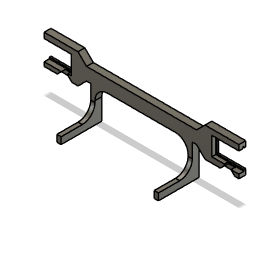
Camera Mount v7 (Autodesk Fusion 360 design; units mm, degrees)
Autodesk Fusion 360 part; units mm, degrees
sketch "Sketch1" plane through (0, 0, 0) normal (0, 0, 1) x (1, 0, 0)
  line L0 (0, 0) -> (-150, 0)
  line L1 (-150, 0) -> (-150, 15)
  line L2 (-150, 15) -> (0, 15)
  line L3 (0, 15) -> (0, 0)
  line L4 (-150, -10) -> (-158, -10)
  line L5 (-158, -10) -> (-158, 25)
  line L6 (-158, 25) -> (-150, 25)
  line L7 (-150, 25) -> (-150, -10)
  line L8 (-158, -5) -> (-188, -5)
  line L9 (-188, -5) -> (-188, 20)
  line L10 (-188, 20) -> (-158, 20)
  line L11 (-158, 20) -> (-158, -5)
  line L12 (-158, -10) -> (-190, -10)
  line L13 (-190, -10) -> (-190, -3.5)
  line L14 (-190, -3.5) -> (-158, -3.5)
  line L15 (-158, -3.5) -> (-158, -10)
  line L16 (-158, 25) -> (-190, 25)
  line L17 (-190, 25) -> (-190, 18.5)
  line L18 (-190, 18.5) -> (-158, 18.5)
  line L19 (-158, 18.5) -> (-158, 25)
  line L20 (0, 25) -> (8, 25)
  line L21 (8, 25) -> (8, -10)
  line L22 (8, -10) -> (0, -10)
  line L23 (0, -10) -> (0, 25)
  line L24 (8, 25) -> (40, 25)
  line L25 (40, 25) -> (40, 18.5)
  line L26 (40, 18.5) -> (8, 18.5)
  line L27 (8, 18.5) -> (8, 25)
  line L28 (8, -10) -> (40, -10)
  line L29 (40, -10) -> (40, -3.5)
  line L30 (40, -3.5) -> (8, -3.5)
  line L31 (8, -3.5) -> (8, -10)
  dimension "d1" = 150
  dimension "d2" = 15
  dimension "d3" = 8
  dimension "d4" = 35
  dimension "d5" = 10
  dimension "d6" = 30
  dimension "d7" = 25
  dimension "d8" = 5
  dimension "d9" = 6.5
  dimension "d10" = 32
  dimension "d11" = 32
  dimension "d12" = 6.5
  dimension "d13" = 8
  dimension "d14" = 35
  dimension "d15" = 10
  dimension "d16" = 32
  dimension "d17" = 6.5
  dimension "d18" = 32
  dimension "d19" = 6.5
  constraint horizontal L0
  constraint vertical L1
  constraint horizontal L2
  constraint vertical L3
  constraint coincident L0.start L3.end
  constraint horizontal L4
  constraint vertical L5
  constraint horizontal L6
  constraint vertical L7
  constraint horizontal L8
  constraint vertical L9
  constraint horizontal L10
  constraint vertical L11
  constraint coincident L5 L8.start
  constraint horizontal L12
  constraint vertical L13
  constraint horizontal L14
  constraint vertical L15
  constraint horizontal L16
  constraint vertical L17
  constraint horizontal L18
  constraint vertical L19
  constraint horizontal L20
  constraint vertical L21
  constraint horizontal L22
  constraint vertical L23
  constraint horizontal L24
  constraint vertical L25
  constraint horizontal L26
  constraint vertical L27
  constraint horizontal L28
  constraint vertical L29
  constraint horizontal L30
  constraint vertical L31
  measures "d1" distance of L0.start L0.end
  measures "d2" distance of L0.end L1.end
  measures "d3" distance of L4.start L4.end
  measures "d4" distance of L4.start L6.end
  measures "d5" distance of L2 L6
  measures "d6" distance of L8.start L8.end
  measures "d7" distance of L8.start L10.end
  measures "d8" distance of L2 L10
  measures "d9" distance of L4.end L14.end
  measures "d10" distance of L4.end L12.end
  measures "d11" distance of L5.end L16.end
  measures "d12" distance of L5.end L18.end
  measures "d13" distance of L20.start L20.end
  measures "d14" distance of L20.start L22.end
  measures "d15" distance of L2 L20
  measures "d16" distance of L20.end L24.end
  measures "d17" distance of L20.end L26.end
  measures "d18" distance of L21.end L28.end
  measures "d19" distance of L21.end L30.end
extrude "Extrude1" add sketch "Sketch1" along normal blind 8 contours L0 L1 L2 L3 L7 L23 | L3 L20 L21 L22 L23 L27 L31 | L1 L4 L5 L6 L7 L11 L15 L19 | L21 L28 L29 L30 L31 | L5 L8 L9 L12 L13 L14 L15 | L21 L24 L25 L26 L27 | L5 L9 L10 L16 L17 L18 L19 | L5 L8 L9 L11 L14 L15 | L5 L9 L10 L11 L18 L19
sketch "Sketch2" plane through (-190, 0, 0) normal (-1, 0, 0) x (0, 0, 1)
  line L0 (0, -3.5) -> (0, -10)
  line L1 (0, -10) -> (8, -10)
  line L2 (8, -10) -> (8, -3.5)
  line L3 (8, -3.5) -> (0, -3.5)
  line L4 (2, -3.5) -> (3.25, -3.5)
  line L5 (3.25, -3.5) -> (3.25, -5.25)
  line L6 (3.25, -5.25) -> (2, -5.25)
  line L7 (2, -5.25) -> (2, -3.5)
  line L8 (2, 18.5) -> (3.25, 18.5)
  line L9 (3.25, 18.5) -> (3.25, 20.25)
  line L10 (3.25, 20.25) -> (2, 20.25)
  line L11 (2, 20.25) -> (2, 18.5)
  dimension "d22" = 1.25
  dimension "d23" = 1.75
  dimension "d24" = 1.25
  dimension "d25" = 1.75
  dimension "d26" = 22
  dimension "d27" = 2
  constraint horizontal L4
  constraint vertical L5
  constraint horizontal L6
  constraint vertical L7
  constraint coincident L3 L4.start
  constraint horizontal L8
  constraint vertical L9
  constraint horizontal L10
  constraint vertical L11
  measures "d22" distance of L4.start L4.end
  measures "d23" distance of L4.start L6.end
  measures "d24" distance of L8.start L8.end
  measures "d25" distance of L8.start L10.end
  measures "d26" distance of L4 L8
  measures "d27" distance of L0 L7
extrude "Extrude2" cut sketch "Sketch2" against normal blind 32 contours L3 L4 L5 L6 L7 | L8 L9 L10 L11
sketch "Sketch3" plane through (-158, 0, 0) normal (-1, 0, 0) x (0, 0, 1)
  line L0 (0, 18.5) -> (0, -3.5)
  line L1 (0, -3.5) -> (2, -3.5)
  line L2 (2, -3.5) -> (2, -5.25)
  line L3 (2, -5.25) -> (3.25, -5.25)
  line L4 (3.25, -5.25) -> (3.25, -3.5)
  line L5 (3.25, -3.5) -> (8, -3.5)
  line L6 (8, -3.5) -> (8, 18.5)
  line L7 (8, 18.5) -> (3.25, 18.5)
  line L8 (3.25, 18.5) -> (3.25, 20.25)
  line L9 (3.25, 20.25) -> (2, 20.25)
  line L10 (2, 20.25) -> (2, 18.5)
  line L11 (2, 18.5) -> (0, 18.5)
  line L12 (2, -5.25) -> (3.25, -5.25)
  line L13 (3.25, -5.25) -> (3.25, 20.25)
  line L14 (3.25, 20.25) -> (2, 20.25)
  line L15 (2, 20.25) -> (2, -5.25)
  constraint horizontal L12
  constraint vertical L13
  constraint horizontal L14
  constraint vertical L15
  constraint coincident L8.end L9.start
  constraint coincident L2.end L3.start
extrude "Extrude3" cut sketch "Sketch3" against normal blind 1.5 contours L2 L3 L4 L8 L9 L10 L12 L13 L14 L15
sketch "Sketch4" plane through (40, 0, 0) normal (1, 0, 0) x (0, 0, -1)
  line L0 (0, -10) -> (0, -3.5)
  line L1 (0, -3.5) -> (-8, -3.5)
  line L2 (-8, -3.5) -> (-8, -10)
  line L3 (-8, -10) -> (0, -10)
  line L4 (-2, -3.5) -> (-3.25, -3.5)
  line L5 (-3.25, -3.5) -> (-3.25, -5.25)
  line L6 (-3.25, -5.25) -> (-2, -5.25)
  line L7 (-2, -5.25) -> (-2, -3.5)
  line L8 (-3.25, 18.5) -> (-2, 18.5)
  line L9 (-2, 18.5) -> (-2, 20.25)
  line L10 (-2, 20.25) -> (-3.25, 20.25)
  line L11 (-3.25, 20.25) -> (-3.25, 18.5)
  line L12 (-2, -5.25) -> (-2, 20.25)
  dimension "d32" = 1.25
  dimension "d33" = 1.75
  dimension "d34" = 2
  dimension "d35" = 1.25
  dimension "d36" = 1.75
  dimension "d37" = 22
  constraint horizontal L4
  constraint vertical L5
  constraint horizontal L6
  constraint vertical L7
  constraint coincident L1 L4.start
  constraint horizontal L8
  constraint vertical L9
  constraint horizontal L10
  constraint vertical L11
  constraint coincident L8.end L12
  measures "d32" distance of L4.start L4.end
  measures "d33" distance of L4.start L6.end
  measures "d34" distance of L0 L7
  measures "d35" distance of L8.start L8.end
  measures "d36" distance of L8.start L10.end
  measures "d37" distance of L4 L8
extrude "Extrude4" cut sketch "Sketch4" against normal blind 32 contours L1 L4 L5 L6 L7 L12 | L8 L9 L10 L11 L12
sketch "Sketch5" plane through (8, 0, 0) normal (1, 0, 0) x (0, 0, -1)
  line L0 (0, -3.5) -> (0, 18.5)
  line L1 (0, 18.5) -> (-2, 18.5)
  line L2 (-2, 18.5) -> (-2, 20.25)
  line L3 (-2, 20.25) -> (-3.25, 20.25)
  line L4 (-3.25, 20.25) -> (-3.25, 18.5)
  line L5 (-3.25, 18.5) -> (-8, 18.5)
  line L6 (-8, 18.5) -> (-8, -3.5)
  line L7 (-8, -3.5) -> (-3.25, -3.5)
  line L8 (-3.25, -3.5) -> (-3.25, -5.25)
  line L9 (-3.25, -5.25) -> (-2, -5.25)
  line L10 (-2, -5.25) -> (-2, -3.5)
  line L11 (-2, -3.5) -> (0, -3.5)
  line L12 (-3.25, 20.25) -> (-2, 20.25)
  line L13 (-2, 20.25) -> (-2, -5.25)
  line L14 (-2, -5.25) -> (-3.25, -5.25)
  line L15 (-3.25, -5.25) -> (-3.25, 20.25)
  constraint horizontal L12
  constraint vertical L13
  constraint horizontal L14
  constraint vertical L15
  constraint coincident L9.end L10.start
  constraint coincident L3.end L4.start
extrude "Extrude5" cut sketch "Sketch5" against normal blind 1.75 contours L2 L3 L4 L8 L9 L10 L12 L13 L14 L15
extrude "Extrude6" cut 1 faces at (-156.5, 11.75, 2.4167) along direction (1, 0, 0) blind 0.25
sketch "Sketch6" plane through (-190, 0, 0) normal (-1, 0, 0) x (0, 0, 1)
  line L0 (2, -5.25) -> (2, -3.5)
  line L1 (2, -3.5) -> (0, -3.5)
  line L2 (0, -3.5) -> (0, -10)
  line L3 (0, -10) -> (8, -10)
  line L4 (8, -10) -> (8, -3.5)
  line L5 (8, -3.5) -> (3.25, -3.5)
  line L6 (3.25, -3.5) -> (3.25, -5.25)
  line L7 (3.25, -5.25) -> (2, -5.25)
  line L8 (3.25, -5.25) -> (8, -5.25)
  line L9 (8, -5.25) -> (8, -3.5)
  line L10 (8, -3.5) -> (3.25, -3.5)
  line L11 (3.25, -3.5) -> (3.25, -5.25)
  constraint horizontal L8
  constraint vertical L9
  constraint horizontal L10
  constraint vertical L11
  constraint coincident L4.end L5.start
  constraint coincident L6.end L7.start
extrude "Extrude7" cut sketch "Sketch6" against normal blind 27.85 contours L4 L5 L6 L8 L9 L10 L11
sketch "Sketch7" plane through (40, 0, 0) normal (1, 0, 0) x (0, 0, -1)
  line L0 (-2, -3.5) -> (-2, -5.25)
  line L1 (-2, -5.25) -> (-3.25, -5.25)
  line L2 (-3.25, -5.25) -> (-3.25, -3.5)
  line L3 (-3.25, -3.5) -> (-8, -3.5)
  line L4 (-8, -3.5) -> (-8, -10)
  line L5 (-8, -10) -> (0, -10)
  line L6 (0, -10) -> (0, -3.5)
  line L7 (0, -3.5) -> (-2, -3.5)
  line L8 (-3.25, -5.25) -> (-8, -5.25)
  line L9 (-8, -5.25) -> (-8, -3.5)
  line L10 (-8, -3.5) -> (-3.25, -3.5)
  line L11 (-3.25, -3.5) -> (-3.25, -5.25)
  constraint horizontal L8
  constraint vertical L9
  constraint horizontal L10
  constraint vertical L11
  constraint coincident L3.end L4.start
  constraint coincident L1.end L2.start
extrude "Extrude8" cut sketch "Sketch7" against normal blind 13.2 contours L2 L3 L4 L8 L9 L10 L11
extrude "Extrude9" cut 1 faces at (26.8, -4.6667, 4.8333) along direction (-1, 0, 0) blind 0.1
extrude "Extrude10" cut 1 faces at (26.7, -4.6667, 4.8333) along direction (-1, 0, 0) blind 0.1
extrude "Extrude11" cut 1 faces at (-162.15, -4.0833, 4.8333) along direction (1, 0, 0) blind 0.1
sketch "Sketch8" plane through (0, -5.25, 0) normal (0, 1, 0) x (-1, 0, 0)
  line L0 (-40, 8) -> (-40, 2)
  line L1 (-40, 2) -> (-6.25, 2)
  line L2 (-6.25, 2) -> (-6.25, 3.25)
  line L3 (-6.25, 3.25) -> (-26.6, 3.25)
  line L4 (-26.6, 3.25) -> (-26.6, 8)
  line L5 (-26.6, 8) -> (-40, 8)
  line L6 (-26.6, 3.25) -> (-34.1, 3.25)
  line L7 (-34.1, 3.25) -> (-34.1, 8)
  line L8 (-34.1, 8) -> (-26.6, 8)
  line L9 (-26.6, 8) -> (-26.6, 3.25)
  dimension "d54" = 7.5
  constraint horizontal L6
  constraint vertical L7
  constraint horizontal L8
  constraint vertical L9
  constraint coincident L3.end L4.start
  constraint coincident L5 L7.end
  measures "d54" distance of L3.end L6.end
extrude "Extrude12" cut sketch "Sketch8" against normal blind 9 contours L4 L5 L6 L7 L8 L9
sketch "Sketch9" plane through (0, -5.25, 0) normal (0, 1, 0) x (-1, 0, 0)
  line L0 (190, 2) -> (190, 8)
  line L1 (190, 8) -> (162.05, 8)
  line L2 (162.05, 8) -> (162.05, 3.25)
  line L3 (162.05, 3.25) -> (156.25, 3.25)
  line L4 (156.25, 3.25) -> (156.25, 2)
  line L5 (156.25, 2) -> (190, 2)
  line L6 (162.05, 3.25) -> (169.55, 3.25)
  line L7 (169.55, 3.25) -> (169.55, 8)
  line L8 (169.55, 8) -> (162.05, 8)
  line L9 (162.05, 8) -> (162.05, 3.25)
  dimension "d57" = 7.5
  constraint horizontal L6
  constraint vertical L7
  constraint horizontal L8
  constraint vertical L9
  constraint coincident L1 L7.end
  constraint coincident L2.end L3.start
  measures "d57" distance of L2.end L6.end
extrude "Extrude13" cut sketch "Sketch9" against normal blind 6 contours L1 L2 L6 L7 L8 L9
extrude "Extrude18" cut 1 faces at (26.6, -6.25, 6.4167) along direction (-1, 0, 0) blind 2
extrude "Extrude19" add 1 faces at (34.1, -6.8333, 4.8333) along direction (-1, 0, 0) blind 2
extrude "Extrude20" cut 1 faces at (24.6, -6.25, 6.4167) along direction (-1, 0, 0) blind 1.75
extrude "Extrude21" add 1 faces at (32.1, -6.8333, 4.8333) along direction (-1, 0, 0) blind 1.75
extrude "Extrude22" cut 1 faces at (30.35, -6.8333, 4.8333) along direction (1, 0, 0) blind 0.2
extrude "Extrude23" cut 1 faces at (-169.55, -6.8333, 4.8333) along direction (-1, 0, 0) blind 0.1
extrude "Extrude24" cut 1 faces at (-162.05, -6.25, 6.4167) along direction (1, 0, 0) blind 0.1
sketch "Sketch14" plane through (0, 0, 8) normal (0, 0, 1) x (1, 0, 0)
  line L0 (-161.95, -3.5) -> (-161.95, -10)
  line L1 (-161.95, -10) -> (-150, -10)
  line L2 (-150, -10) -> (-150, 0)
  line L3 (-150, 0) -> (0, 0)
  line L4 (0, 0) -> (0, -10)
  line L5 (0, -10) -> (22.85, -10)
  line L6 (22.85, -10) -> (22.85, -3.5)
  line L7 (22.85, -3.5) -> (8, -3.5)
  line L8 (8, -3.5) -> (8, 18.5)
  line L9 (8, 18.5) -> (40, 18.5)
  line L10 (40, 18.5) -> (40, 25)
  line L11 (40, 25) -> (0, 25)
  line L12 (0, 25) -> (0, 15)
  line L13 (0, 15) -> (-150, 15)
  line L14 (-150, 15) -> (-150, 25)
  line L15 (-150, 25) -> (-190, 25)
  line L16 (-190, 25) -> (-190, 18.5)
  line L17 (-190, 18.5) -> (-158, 18.5)
  line L18 (-158, 18.5) -> (-158, -3.5)
  line L19 (-158, -3.5) -> (-161.95, -3.5)
  line L20 (22.85, -5.25) -> (22.85, -10)
  line L21 (22.85, -10) -> (18.1, -10)
  line L22 (22.85, -5.25) -> (18.1, -10)
  dimension "d89" = 4.75
  dimension "d90" = 4.75
  constraint coincident L6 L20.start
  constraint coincident L5.end L6.start
  constraint perpendicular L5 L20
  constraint perpendicular L6 L21
  measures "d89" distance of L20.start L5.end
  measures "d90" distance of L5.end L21.end
extrude "Extrude25" cut sketch "Sketch14" against normal blind 4.75 contours L5 L6 L20 L21 L22
sketch "Sketch15" plane through (0, 0, 8) normal (0, 0, 1) x (1, 0, 0)
  line L0 (30.55, -5.25) -> (30.55, -10)
  line L1 (30.55, -10) -> (40, -10)
  line L2 (40, -10) -> (40, -5.25)
  line L3 (40, -5.25) -> (30.55, -5.25)
  line L4 (30.55, -5.25) -> (30.55, -10)
  line L5 (30.55, -10) -> (35.3, -10)
  line L6 (30.55, -5.25) -> (35.3, -10)
  dimension "d93" = 4.75
  constraint coincident L0.start L3.end
  constraint coincident L0.end L1.start
  constraint perpendicular L0 L5
  measures "d93" distance of L0.end L5.end
extrude "Extrude26" cut sketch "Sketch15" against normal blind 4.75 contours L0 L1 L4 L5 L6
sketch "Sketch16" plane through (0, 0, 8) normal (0, 0, 1) x (1, 0, 0)
  line L0 (-169.65, -10) -> (-169.65, -5.25)
  line L1 (-169.65, -5.25) -> (-190, -5.25)
  line L2 (-190, -5.25) -> (-190, -10)
  line L3 (-190, -10) -> (-169.65, -10)
  line L4 (-169.65, -5.25) -> (-169.65, -10)
  line L5 (-169.65, -10) -> (-174.4, -10)
  line L6 (-174.4, -10) -> (-169.65, -5.25)
  dimension "d60" = 4.75
  dimension "d61" = 4.75
  dimension "d96" = 4.75
  constraint coincident L0.end L1.start
  constraint coincident L0.start L3.end
  constraint perpendicular L4 L5
  measures "d96" distance of L0.start L5.end
extrude "Extrude27" cut sketch "Sketch16" against normal blind 4.75 contours L0 L3 L4 L5 L6
sketch "Sketch17" plane through (0, 0, 8) normal (0, 0, 1) x (1, 0, 0)
  line L0 (18.1, -10) -> (22.85, -5.25)
  line L1 (22.85, -5.25) -> (22.85, -3.5)
  line L2 (22.85, -3.5) -> (8, -3.5)
  line L3 (8, -3.5) -> (8, 18.5)
  line L4 (8, 18.5) -> (40, 18.5)
  line L5 (40, 18.5) -> (40, 25)
  line L6 (40, 25) -> (0, 25)
  line L7 (0, 25) -> (0, 15)
  line L8 (0, 15) -> (-150, 15)
  line L9 (-150, 15) -> (-150, 25)
  line L10 (-150, 25) -> (-190, 25)
  line L11 (-190, 25) -> (-190, 18.5)
  line L12 (-190, 18.5) -> (-158, 18.5)
  line L13 (-158, 18.5) -> (-158, -3.5)
  line L14 (-158, -3.5) -> (-161.95, -3.5)
  line L15 (-161.95, -3.5) -> (-161.95, -10)
  line L16 (-161.95, -10) -> (-150, -10)
  line L17 (-150, -10) -> (-150, 0)
  line L18 (-150, 0) -> (0, 0)
  line L19 (0, 0) -> (0, -10)
  line L20 (0, -10) -> (18.1, -10)
  line L21 (-161.95, -10) -> (-161.95, -5.25)
  line L22 (-161.95, -10) -> (-157.2, -10)
  line L23 (-161.95, -5.25) -> (-157.2, -10)
  dimension "d99" = 4.75
  dimension "d100" = 4.75
  constraint coincident L15.end L16.start
  constraint perpendicular L16 L21
  constraint perpendicular L15 L22
  measures "d99" distance of L15.end L21.end
  measures "d100" distance of L15.end L22.end
extrude "Extrude28" cut sketch "Sketch17" against normal blind 4.75 contours L15 L16 L21 L22 L23
sketch "Sketch18" plane through (0, 0, 8) normal (0, 0, 1) x (1, 0, 0)
  line L0 (-161.95, -5.25) -> (-157.2, -10)
  line L1 (-157.2, -10) -> (-150, -10)
  line L2 (-150, -10) -> (-150, 0)
  line L3 (-150, 0) -> (0, 0)
  line L4 (0, 0) -> (0, -10)
  line L5 (0, -10) -> (18.1, -10)
  line L6 (18.1, -10) -> (22.85, -5.25)
  line L7 (22.85, -5.25) -> (22.85, -3.5)
  line L8 (22.85, -3.5) -> (8, -3.5)
  line L9 (8, -3.5) -> (8, 18.5)
  line L10 (8, 18.5) -> (40, 18.5)
  line L11 (40, 18.5) -> (40, 25)
  line L12 (40, 25) -> (0, 25)
  line L13 (0, 25) -> (0, 15)
  line L14 (0, 15) -> (-150, 15)
  line L15 (-150, 15) -> (-150, 25)
  line L16 (-150, 25) -> (-190, 25)
  line L17 (-190, 25) -> (-190, 18.5)
  line L18 (-190, 18.5) -> (-158, 18.5)
  line L19 (-158, 18.5) -> (-158, -3.5)
  line L20 (-158, -3.5) -> (-161.95, -3.5)
  line L21 (-161.95, -3.5) -> (-161.95, -5.25)
  line L22 (0, 25) -> (0, 15)
  line L23 (0, 15) -> (-10, 15)
  line L24 (-10, 15) -> (0, 25)
  line L25 (0, 0) -> (-10, 0)
  line L26 (0, 0) -> (0, -10)
  line L27 (0, -10) -> (-10, 0)
  line L28 (-150, 25) -> (-150, 15)
  line L29 (-150, 15) -> (-140, 15)
  line L30 (-150, 25) -> (-140, 15)
  line L31 (-150, 0) -> (-150, -10)
  line L32 (-150, 0) -> (-140, 0)
  line L33 (-150, -10) -> (-140, 0)
  dimension "d103" = 10
  dimension "d104" = 10
  dimension "d105" = 10
  dimension "d106" = 10
  constraint coincident L12.end L13.start
  constraint coincident L13.end L14.start
  constraint perpendicular L13 L23
  constraint coincident L3.end L4.start
  constraint perpendicular L4 L25
  constraint coincident L4.end L5.start
  constraint coincident L15.end L16.start
  constraint coincident L14.end L15.start
  constraint perpendicular L15 L29
  constraint coincident L2.end L3.start
  constraint coincident L1.end L2.start
  constraint perpendicular L2 L32
  measures "d103" distance of L13.end L23.end
  measures "d104" distance of L3.end L25.end
  measures "d105" distance of L14.end L29.end
  measures "d106" distance of L2.end L32.end
extrude "Extrude29" add sketch "Sketch18" against normal blind 8 contours L2 L3 L31 L32 L33 | L3 L4 L25 L26 L27 | L14 L15 L28 L29 L30 | L13 L14 L22 L23 L24
sketch "Sketch19" plane through (0, 0, 8) normal (0, 0, 1) x (1, 0, 0)
  line L0 (-161.95, -5.25) -> (-157.2, -10)
  line L1 (-157.2, -10) -> (-150, -10)
  line L2 (-150, -10) -> (-140, 0)
  line L3 (-140, 0) -> (-10, 0)
  line L4 (-10, 0) -> (0, -10)
  line L5 (0, -10) -> (18.1, -10)
  line L6 (18.1, -10) -> (22.85, -5.25)
  line L7 (22.85, -5.25) -> (22.85, -3.5)
  line L8 (22.85, -3.5) -> (8, -3.5)
  line L9 (8, -3.5) -> (8, 18.5)
  line L10 (8, 18.5) -> (40, 18.5)
  line L11 (40, 18.5) -> (40, 25)
  line L12 (40, 25) -> (0, 25)
  line L13 (0, 25) -> (-10, 15)
  line L14 (-10, 15) -> (-140, 15)
  line L15 (-140, 15) -> (-150, 25)
  line L16 (-150, 25) -> (-190, 25)
  line L17 (-190, 25) -> (-190, 18.5)
  line L18 (-190, 18.5) -> (-158, 18.5)
  line L19 (-158, 18.5) -> (-158, -3.5)
  line L20 (-158, -3.5) -> (-161.95, -3.5)
  line L21 (-161.95, -3.5) -> (-161.95, -5.25)
  line L22 (-135, 0) -> (-130, 0)
  line L23 (-130, 0) -> (-130, -40)
  line L24 (-130, -40) -> (-135, -40)
  line L25 (-135, -40) -> (-135, 0)
  line L26 (-15, 0) -> (-20, 0)
  line L27 (-20, 0) -> (-20, -40)
  line L28 (-20, -40) -> (-15, -40)
  line L29 (-15, -40) -> (-15, 0)
  dimension "d109" = 40
  dimension "d110" = 40
  constraint horizontal L22
  constraint vertical L23
  constraint horizontal L24
  constraint vertical L25
  constraint coincident L3 L22.start
  constraint horizontal L26
  constraint vertical L27
  constraint horizontal L28
  constraint vertical L29
  constraint coincident L3 L26.start
  measures "d109" distance of L22.start L24.end
  measures "d110" distance of L26.start L28.end
extrude "Extrude30" add sketch "Sketch19" against normal blind 8 contours L3 L22 L23 L24 L25 | L3 L26 L27 L28 L29
sketch "Sketch20" plane through (0, 0, 8) normal (0, 0, 1) x (1, 0, 0)
  line L0 (-161.95, -5.25) -> (-157.2, -10)
  line L1 (-157.2, -10) -> (-150, -10)
  line L2 (-150, -10) -> (-140, 0)
  line L3 (-140, 0) -> (-135, 0)
  line L4 (-135, 0) -> (-135, -40)
  line L5 (-135, -40) -> (-130, -40)
  line L6 (-130, -40) -> (-130, 0)
  line L7 (-130, 0) -> (-20, 0)
  line L8 (-20, 0) -> (-20, -40)
  line L9 (-20, -40) -> (-15, -40)
  line L10 (-15, -40) -> (-15, 0)
  line L11 (-15, 0) -> (-10, 0)
  line L12 (-10, 0) -> (0, -10)
  line L13 (0, -10) -> (18.1, -10)
  line L14 (18.1, -10) -> (22.85, -5.25)
  line L15 (22.85, -5.25) -> (22.85, -3.5)
  line L16 (22.85, -3.5) -> (8, -3.5)
  line L17 (8, -3.5) -> (8, 18.5)
  line L18 (8, 18.5) -> (40, 18.5)
  line L19 (40, 18.5) -> (40, 25)
  line L20 (40, 25) -> (0, 25)
  line L21 (0, 25) -> (-10, 15)
  line L22 (-10, 15) -> (-140, 15)
  line L23 (-140, 15) -> (-150, 25)
  line L24 (-150, 25) -> (-190, 25)
  line L25 (-190, 25) -> (-190, 18.5)
  line L26 (-190, 18.5) -> (-158, 18.5)
  line L27 (-158, 18.5) -> (-158, -3.5)
  line L28 (-158, -3.5) -> (-161.95, -3.5)
  line L29 (-161.95, -3.5) -> (-161.95, -5.25)
  line L30 (-135, -40) -> (-130, -40)
  line L31 (-130, -40) -> (-130, -35)
  line L32 (-130, -35) -> (-135, -35)
  line L33 (-135, -35) -> (-135, -40)
  line L34 (-20, -40) -> (-15, -40)
  line L35 (-15, -40) -> (-15, -35)
  line L36 (-15, -35) -> (-20, -35)
  line L37 (-20, -35) -> (-20, -40)
  constraint horizontal L30
  constraint vertical L31
  constraint horizontal L32
  constraint vertical L33
  constraint coincident L6 L31.end
  constraint coincident L4.end L5.start
  constraint horizontal L34
  constraint vertical L35
  constraint horizontal L36
  constraint vertical L37
  constraint coincident L10 L35.end
  constraint coincident L8.end L9.start
extrude "Extrude31" add sketch "Sketch20" along normal blind 40 contours L4 L5 L6 L30 L31 L32 L33 | L8 L9 L10 L34 L35 L36 L37
extrude "Extrude32" add 2 faces at (-16.6667, -35, 34.6667) (-131.6667, -35, 21.3333) along direction (0, 1, 0) blind 3
fillet "Fillet1" radius 15 2 edges at (-132.5, -32, 8) (-17.5, -32, 8)
fillet "Fillet2" radius 15 2 edges at (-20, 0, 4) (-130, 0, 4)
